Autodesk Inventor part; units mm, degrees
(part 2 of 2)
sketch "Sketch8" plane through (0, 0, 0) normal (0, 0, 1) x (1, 0, 0)
  line L0 (7.5, -1.5) -> (-7.5, -1.5) construction
  circle A0 centre (0, -1.5) radius 16.5 construction
  line L1 (21, -1.5) -> (-21, -1.5) construction
  line L2 (16.5, -1.5) -> (-16.5, -1.5) construction
  line L3 (-16.5, -1.5) -> (-16.5, 15) construction
  line L4 (-16.5, 15) -> (16.5, 15) construction
  line L5 (16.5, 15) -> (16.5, -1.5) construction
  circle A1 centre (0, 15) radius 1.575
  point P0 (0, 0)
  dimension "d23" = 33
  dimension "d24" = 33
  dimension "d25" = 16.5
  dimension "d26" = 3.15
  constraints: 8 end point, 2 midpoint, 2 parallel, 1 centre point, 1 horizontal, 1 horizontal alignment, 1 perpendicular, 1 point on line, 2 other
  measures "d24" distance of L3.end L4.end
  measures "d25" distance of L2.end L3.end
  measures "d26" diameter of A1
extrude "Extrusion2" cut sketch "Sketch8" against normal blind 30
ref_plane "Work Plane3" through (0, 0, -16.75) normal (0, 0, 1) x (1, 0, 0)
sketch "Sketch10" plane through (0, 0, -16.75) normal (0, 0, 1) x (1, 0, 0)
  line L0 (-0.0163, 0) -> (-0.0163, 30) projected
  circle A0 centre (-0.0163, 15) radius 3
  point P0 (0, 0)
  dimension "d30" = 6
  constraints: 1 centre point, 1 midpoint
  measures "d30" diameter of A0
extrude "Extrusion3" cut sketch "Sketch10" along normal blind 4 and the other way blind 2.5
sketch "Sketch11" plane through (0, 0, 0) normal (1, 0, 0) x (0, 1, 0)
  line L0 (-1.5, -7.5) -> (-1.5, 7.5) projected
  circle A0 centre (-1.5, 0) radius 16.5 construction
  line L1 (-1.5, -16.5) -> (15, -16.5)
  line L2 (15, -16.5) -> (15, 16.5)
  line L3 (15, 16.5) -> (-1.5, 16.5)
  line L4 (-1.5, 16.5) -> (-1.5, -16.5)
  line L5 (0, -0.0002) -> (30, -0.0002) projected
  circle A1 centre (15, -0.0002) radius 1.575
  point P0 (0, 0)
  dimension "d35" = 33
  dimension "d36" = 16.5
  dimension "d37" = 33
  dimension "d38" = 3.15
  constraints: 8 end point, 2 midpoint, 2 parallel, 1 centre point, 1 horizontal, 1 perpendicular, 1 vertical alignment, 2 other
  measures "d36" distance of L3.end L2.end
  measures "d37" distance of L2.end L1.end
  measures "d38" diameter of A1
extrude "Extrusion4" cut sketch "Sketch11" against normal through all contours A1 L5 L2 | L2 L5 A1 | A1 L5 L2 | L2 L5 A1
ref_plane "Work Plane4" through (-16.5, 0, 0) normal (1, 0, 0) x (0, 1, 0)
sketch "Sketch12" plane through (-16.5, 0, 0) normal (1, 0, 0) x (0, 1, 0)
  line L0 (0, -0.0002) -> (30, -0.0002) projected
  circle A0 centre (15, -0.0002) radius 3
  point P0 (0, 0)
  dimension "d42" = 6
  constraints: 1 centre point, 1 midpoint
  measures "d42" diameter of A0
extrude "Extrusion5" cut sketch "Sketch12" along normal blind 3 and the other way blind 5
sketch "Sketch13" plane through (0, -1.5, 0) normal (0, -1, 0) x (1, 0, 0)
  point P0 (0, 0)
ref_plane "Work Plane5" through (0, 0, -8.375) normal (0, 0, 1) x (1, 0, 0)
sketch "Sketch14" plane through (0, 0, -8.375) normal (0, 0, 1) x (1, 0, 0)
  line L0 (0, 11.5359) -> (-3, 13.2679)
  line L1 (-3, 13.2679) -> (-3, 16.7321)
  line L2 (-3, 16.7321) -> (0, 18.4641)
  line L3 (0, 18.4641) -> (3, 16.7321)
  line L4 (3, 16.7321) -> (3, 13.2679)
  line L5 (3, 13.2679) -> (0, 11.5359)
  line L6 (3, 13.2679) -> (-3, 13.2679)
  line L7 (-3, 13.2679) -> (-3, -1.7321)
  line L8 (-3, -1.7321) -> (3, -1.7321)
  line L9 (3, -1.7321) -> (3, 13.2679)
  point P0 (0, 0)
  point P1 (0, 15)
  dimension "d47" = 6
  dimension "d48" = 6
  dimension "d49" = 15
  constraints: 20 end point, 2 parallel, 1 horizontal, 1 perpendicular, 13 other
  measures "d47" distance between parallel lines of L1 L4
  measures "d48" distance of L8.end L7.end
  measures "d49" distance of L7.end L6.end
extrude "Extrusion6" cut sketch "Sketch14" against normal blind 2.35
ref_plane "Work Plane6" through (-8.25, 0, 0) normal (1, 0, 0) x (0, 1, 0)
sketch "Sketch15" plane through (-8.25, 0, 0) normal (1, 0, 0) x (0, 1, 0)
  line L0 (0, -0.0002) -> (30, -0.0002) projected
  line L1 (11.5359, -0.0002) -> (13.2679, 2.9998)
  line L2 (13.2679, 2.9998) -> (16.7321, 2.9998)
  line L3 (16.7321, 2.9998) -> (18.4641, -0.0002)
  line L4 (18.4641, -0.0002) -> (16.7321, -3.0002)
  line L5 (16.7321, -3.0002) -> (13.2679, -3.0002)
  line L6 (13.2679, -3.0002) -> (11.5359, -0.0002)
  line L7 (13.2679, -3.0002) -> (-1.7321, -3.0002)
  line L8 (-1.7321, -3.0002) -> (-1.7321, 2.9998)
  line L9 (-1.7321, 2.9998) -> (13.2679, 2.9998)
  line L10 (13.2679, 2.9998) -> (13.2679, -3.0002)
  point P0 (0, 0)
  point P1 (15, -0.0002)
  dimension "d52" = 6
  dimension "d53" = 15
  dimension "d54" = 6
  constraints: 20 end point, 2 parallel, 1 horizontal, 1 midpoint, 1 perpendicular, 1 point on line, 13 other
  measures "d52" distance between parallel lines of L2 L5
  measures "d53" distance of L8.end L9.end
  measures "d54" distance of L7.end L8.end
extrude "Extrusion7" cut sketch "Sketch15" against normal blind 2.35
body "Solid1"
